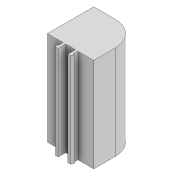
# Autodesk Inventor part: Blank
Saved by Autodesk Inventor 2021 (Build 250183000, 183)
## iProperties
Created: 2021-07-29
Part Number: Blank
Material: Generisch
Document SubType Name: Modeling
Designer: Rama
Density: 1 g/cm^3
Appearance: Vorgabe
Author: Rama
Autodesk Inventor part; units mm, degrees
ref_plane "YZ Plane" through (0, 0, 0) normal (1, 0, 0) x (0, 1, 0)
ref_plane "XZ Plane" through (0, 0, 0) normal (0, 1, 0) x (-1, 0, 0)
ref_plane "XY Plane" through (0, 0, 0) normal (0, 0, 1) x (1, 0, 0)
sketch "Skizze1" plane through (0, 0, 0) normal (0, 1, 0) x (-1, 0, 0)
  line L0 (10, 10) -> (-10, 10)
  line L1 (-10, 10) -> (-10, -10)
  line L2 (-10, -10) -> (10, -10)
  line L3 (10, -10) -> (10, 10)
  line L4 (10, 10) -> (-10, -10) construction
  line L5 (-10, 10) -> (10, -10) construction
  point P0 (0, 0)
  dimension "d0" = 20
  dimension "d1" = 20
  constraints: 12 end point, 2 midpoint, 2 parallel, 1 horizontal, 1 perpendicular
  measures "d0" distance of L2.end L1.end
  measures "d1" distance of L1.end L0.end
extrude "Extrusion1" add sketch "Skizze1" along normal blind 34.5
sketch "Skizze2" plane through (0, 0, 0) normal (0, -1, 0) x (1, 0, 0)
  line L0 (-8.9654, -8) -> (-1.6431, -8)
  line L1 (8, 1.6431) -> (8, 9.2)
  line L2 (-10, 10) -> (10, 10)
  line L3 (-10, -10) -> (-10, 10)
  line L4 (8, 10) -> (-10, 10)
  line L5 (-10, 10) -> (-10, -8)
  line L6 (-10, -8) -> (8, -8)
  line L7 (8, -8) -> (8, 10)
  line L8 (10, 10) -> (10, -10)
  line L9 (-10, 10) -> (10, 10)
  line L10 (-10, -10) -> (-10, 10)
  line L11 (10, -10) -> (-10, -10)
  circle A0 centre (-1.6431, 1.6431) radius 9.6431
  point P0 (0, 0)
  constraints: 24 end point, 2 point on line, 3 other
extrude "Extrusion2" cut sketch "Skizze2" against normal through all contours L0 L6 L7 L1 L2 L8 L11 L3 | A0 L7 L6
sketch "Skizze3" plane through (0, 34.5, 0) normal (0, 1, 0) x (1, 0, 0)
  line L0 (0.9, -9.6) -> (0.9, -12.8936) projected
  line L1 (0.9, -12.8936) -> (1.9, -12.8936) projected
  line L2 (1.9, -12.8936) -> (2.4, -11.85) projected
  line L3 (2.4, -11.85) -> (1.9, -11.85) projected
  line L4 (1.9, -12.8936) -> (1.9, -9.6) projected
  line L5 (-2.9, -12.8936) -> (-2.9, -9.6) projected
  line L6 (-3.9, -9.6) -> (-3.9, -12.8936) projected
  line L7 (-3.9, -11.85) -> (-4.4, -11.85) projected
  line L8 (-4.4, -11.85) -> (-3.9, -12.8936) projected
  line L9 (-3.9, -12.8936) -> (-2.9, -12.8936) projected
  line L10 (0.9, -12.8936) -> (1.9, -12.8936)
  line L11 (1.9, -12.8936) -> (1.9, -9.6)
  line L12 (1.9, -9.6) -> (0.9, -9.6)
  line L13 (0.9, -9.6) -> (0.9, -12.8936)
  line L14 (-2.9, -12.8936) -> (-3.9, -12.8936)
  line L15 (-3.9, -12.8936) -> (-3.9, -9.6)
  line L16 (-3.9, -9.6) -> (-2.9, -9.6)
  line L17 (-2.9, -9.6) -> (-2.9, -12.8936)
  point P0 (0, 0)
  constraints: 16 end point, 4 parallel, 2 horizontal, 2 perpendicular
extrude "Extrusion3" add sketch "Skizze3" against normal up to surface (34.5 mm away)
move faces "Verschieben1" translate (0, 2, 0) faces at (-5.181, 34.5, -2)
